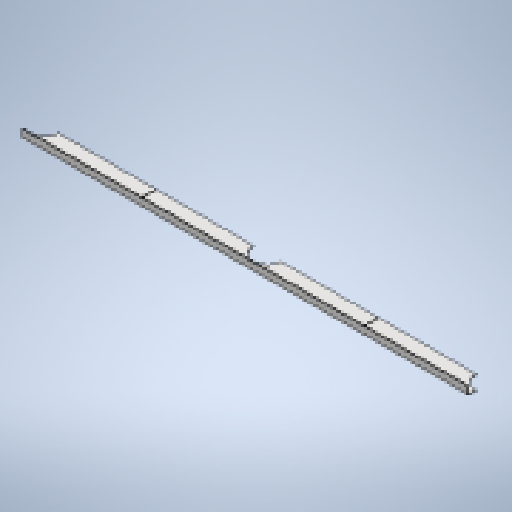
# Autodesk Inventor part: MSC 504 STRINGER BOARD BELLY
Saved by Autodesk Inventor 2025 (Build 290162010, 162A)
## iProperties
Created: 2024-04-28
Part Number: MSC 504 STRINGER BOARD BELLY
Material: Stainless Steel
Document SubType Name: Sheet Metal
Designer: pokla
Density: 8 g/cm^3
Flat Pattern Width: 6.6202 cm
Flat Pattern Length: 98 cm
Flat Pattern Area: 648.78 cm^2
Sheet Metal Rule: AISI304 2mm Die16
Sheet Metal Width: 66,202 mm
Sheet Metal Length: 980,000 mm
Sheet Metal Area: 64877,951 mm^2
Appearance: Default
Stock Number: МОО 504 стрингер борт живот
Author: admin
Autodesk Inventor part; units mm, degrees
ref_plane "YZ Plane" through (0, 0, 0) normal (1, 0, 0) x (0, 1, 0)
ref_plane "XZ Plane" through (0, 0, 0) normal (0, 1, 0) x (-1, 0, 0)
ref_plane "XY Plane" through (0, 0, 0) normal (0, 0, 1) x (1, 0, 0)
sketch "Sketch1" plane through (0, 0, 0) normal (0, 0, 1) x (1, 0, 0)
  line L0 (-490, 50) -> (490, 50)
  line L1 (490, 50) -> (490, 0)
  line L2 (490, 0) -> (-490, 0)
  line L3 (-490, 0) -> (-490, 50)
  point P0 (0, 0)
  point P1 (0, 0)
  dimension "d0" = 980
  dimension "d1" = 50
  measures "d0" distance of L1.end L2.end
  measures "d1" distance of L0.end L1.end
extrude "Plate1" add sketch "Sketch1" along normal blind 2
sketch "Sketch2" plane through (490, 2, 0) normal (0, -1, 0) x (1, 0, 0)
  line L0 (-980, 0) -> (0, 0)
  line L1 (0, 0) -> (0, 20)
  line L2 (0, 20) -> (-980, 20)
  line L3 (-980, 20) -> (-980, 0)
  constraints: 6 end point, 1 horizontal, 1 perpendicular, 1 vertical
edge flange "Flange1" height 20 angle 90 thickness 2 bend radius 2.75 thickness toward (0, -1, 0) relief straight relief width 2 relief depth 1 edges at (0, 0, 2) wall of the first edge with corners at (-490, 2, 0) (490, 2, 0) (490, 2, 20) (-490, 2, 20)
bend "Bend1"
corner "Corner1"
sketch "Sketch5" plane through (0, 0, 0) normal (0, 0, -1) x (-1, 0, 0)
  line L0 (490, 50) -> (-490, 50) projected
  line L1 (490, 0) -> (-490, 0) projected
  circle A0 centre (0, 50) radius 30
  line L2 (-490, 0) -> (-490, 50)
  line L3 (490, 0) -> (490, 50)
  circle A1 centre (-490, 50) radius 30
  circle A2 centre (490, 50) radius 30
  line L4 (-246, 50) -> (-244, 50)
  line L5 (-244, 50) -> (-244, 19)
  line L6 (-244, 19) -> (-246, 19)
  line L7 (-246, 19) -> (-246, 50)
  line L8 (244, 50) -> (246, 50)
  line L9 (246, 50) -> (246, 19)
  line L10 (246, 19) -> (244, 19)
  line L11 (244, 19) -> (244, 50)
  line L12 (0, 50) -> (0, 0) construction
  point P0 (245, 19)
  point P1 (-245, 19)
  point P2 (-490, 20)
  point P3 (-460, 50)
  point P4 (-30, 50)
  point P5 (30, 50)
  point P6 (460, 50)
  point P7 (490, 20)
  point P8 (-244, 50)
  point P9 (246, 50)
  dimension "d33" = 60
  dimension "d34" = 2
  dimension "d35" = 31
  dimension "d36" = 490
  constraints: 22 end point, 5 parallel, 4 midpoint, 3 centre point, 3 point on line, 2 coincident, 2 equal radius, 2 horizontal, 2 perpendicular, 1 collinear, 1 vertical, 1 other
  measures "d33" diameter of A0
  measures "d34" distance of L5.end L6.end
  measures "d35" distance of L4.end L5.end
  measures "d36" distance of point (245, 19) point (-245, 19)
extrude "Extrusion1" cut sketch "Sketch5" against normal through all contours L9 L10 L11 L0 | L0 L3 A2 | A0 L0 | L5 L6 L7 L0 | L2 L0 A1 picked at (470.2507, 47.7748) picked at (6.5355, 34.7298) picked at (-470.2507, 47.7748)
sketch "Sketch7" plane through (0, 0, 2) normal (0, 0, 1) x (1, 0, 0)
  line L0 (468.7934, 20.88) -> (468.7934, 8.88) construction
  line L1 (468.7934, 8.88) -> (251.3453, 8.88) construction
  line L2 (251.3453, 8.88) -> (251.3453, 20.88) construction
  line L3 (251.3453, 20.88) -> (468.7934, 20.88) construction
  line L4 (-244, 50) -> (-30, 50) projected
  point P0 (0, 0)
  point P1 (-1, 50)
  point P2 (1, 50)
  dimension "d30" = 12
  constraints: 2 other
  measures "d30" distance of L2.start L2.end
mark "Mark1"
equation "\"d1\" = Стрингер_7"
equation "\"d2\" = Thickness"
equation "\"d3\" = BendReliefWidth"
equation "\"d4\" = BendReliefDepth"
equation "\"d5\" = MinimumRemnant"
equation "\"d6\" = TransitionRadius"
equation "\"d9\" = BendRadius"
equation "\"d10\" = CornerReliefSize"
equation "\"d11\" = GapSize"
equation "\"d12\" = JacobiRadiusSize"
equation "\"GapSize\" = Thickness"
equation "\"MinimumRemnant\" = 2 * Thickness"
equation "\"BendReliefDepth\" = 0.5 * Thickness"
equation "\"BendReliefWidth\" = Thickness"
equation "\"CornerReliefSize\" = 4 * Thickness"
equation "\"JacobiRadiusSize\" = BendRadius"
equation "\"TransitionRadius\" = BendRadius"
equation "\"Стрингер_7\" = 50"
equation "\"Thickness\" = 2"
equation "\"BendRadius\" = 2.75"
body "Solid1"
